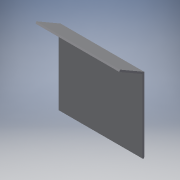
# Autodesk Inventor part: flap
Saved by Autodesk Inventor 2017 (Build 210142000, 142)
## iProperties
Created: 2019-01-31
Part Number: flap
Material: Generic
Document SubType Name: Modeling
Designer: S346553810
Density: 1 g/cm^3
Appearance: Default
Author: S346553810
Autodesk Inventor part; units mm, degrees
ref_plane "YZ Plane" through (0, 0, 0) normal (1, 0, 0) x (0, 1, 0)
ref_plane "XZ Plane" through (0, 0, 0) normal (0, 1, 0) x (-1, 0, 0)
ref_plane "XY Plane" through (0, 0, 0) normal (0, 0, 1) x (1, 0, 0)
sketch "Sketch6" plane through (0, 0, 0) normal (0, 1, 0) x (-1, 0, 0)
  line L0 (0, 0) -> (43.9941, -25.4)
  line L1 (43.9941, -25.4) -> (43.9941, -158.75)
  line L2 (43.9941, -158.75) -> (44.6063, -159.1035)
  line L3 (43.9941, -158.75) -> (44.701, -158.75) construction
  line L4 (43.0188, -161.8531) -> (40.8191, -160.5831)
  line L5 (40.8191, -160.5831) -> (40.8191, -27.2331)
  line L6 (40.8191, -27.2331) -> (-1.5875, -2.7496)
  line L7 (-1.5875, -2.7496) -> (0, 0)
  line L8 (0, 0) -> (22.7499, 0) construction
  line L9 (43.0188, -161.8531) -> (44.6063, -159.1035)
  dimension "d15" = 50.8
  dimension "d17" = 133.35
  dimension "d21" = 3.175
  dimension "d22" = 30
  dimension "d27" = 120
  dimension "d29" = 2.54
  dimension "d30" = 90
  constraints: 20 end point, 2 horizontal, 1 equal length, 1 vertical, 2 other
  measures "d15" distance of L0.start L0.end
  measures "d17" distance of L0.end L1.end
  measures "d21" distance between parallel lines of L1 L5
  measures "d22" angle of L8 L0
  measures "d27" angle of L1 L2
  measures "d29" distance of L4.start L4.end
  measures "d30" angle of L4 L9
extrude "Extrusion5" add sketch "Sketch6" along normal blind 152.4
body "Solid2"
